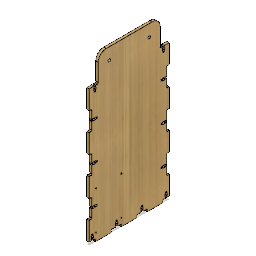
Square-plate-IIIS-power-rev1_8mm v1 (Autodesk Fusion 360 design; units mm, degrees)
Autodesk Fusion 360 part; units mm, degrees
sketch "Basic shape" plane through (0, 0, 0) normal (1, 0, 0) x (0, 0, -1)
  line L0 (-117.75, 0) -> (117.75, 0)
  line L1 (117.75, 0) -> (117.75, 417)
  line L2 (117.75, 417) -> (-117.75, 417)
  line L3 (-117.75, 417) -> (-117.75, 0)
  line L4 (-97.5, 417) -> (97.5, 417)
  line L5 (97.5, 417) -> (97.5, 500)
  line L6 (97.5, 500) -> (-97.5, 500)
  line L7 (-97.5, 500) -> (-97.5, 417)
  line L8 (117.75, 0) -> (125.75, 0)
  line L9 (125.75, 0) -> (125.75, 60)
  line L10 (125.75, 60) -> (117.75, 60)
  line L11 (117.75, 60) -> (117.75, 0)
  line L12 (117.75, 119) -> (125.75, 119)
  line L13 (125.75, 119) -> (125.75, 179)
  line L14 (125.75, 179) -> (117.75, 179)
  line L15 (117.75, 179) -> (117.75, 119)
  line L16 (117.75, 238) -> (125.75, 238)
  line L17 (125.75, 238) -> (125.75, 298)
  line L18 (125.75, 298) -> (117.75, 298)
  line L19 (117.75, 298) -> (117.75, 238)
  line L20 (117.75, 357) -> (125.75, 357)
  line L21 (125.75, 357) -> (125.75, 417)
  line L22 (125.75, 417) -> (117.75, 417)
  line L23 (117.75, 417) -> (117.75, 357)
  curve K0
  line L24 (-55.75, 0) -> (-55.75, -8)
  line L25 (-55.75, -8) -> (-105.75, -8)
  line L26 (-25, 0) -> (25, 0)
  line L27 (25, 0) -> (25, -8)
  line L28 (25, -8) -> (-25, -8)
  line L29 (-25, -8) -> (-25, 0)
  line L30 (117.75, 0) -> (55.75, 0)
  line L31 (55.75, 0) -> (55.75, -8)
  line L32 (55.75, -8) -> (105.75, -8)
  line L33 (-55.75, -8) -> (-25, -8) construction
  line L34 (25, -8) -> (55.75, -8) construction
  line L35 (-117.75, 0) -> (-125.75, 0)
  line L36 (-125.75, 0) -> (-125.75, 60)
  line L37 (-125.75, 60) -> (-117.75, 60)
  line L38 (-117.75, 60) -> (-117.75, 0)
  line L39 (-117.75, 119) -> (-125.75, 119)
  line L40 (-125.75, 119) -> (-125.75, 179)
  line L41 (-125.75, 179) -> (-117.75, 179)
  line L42 (-117.75, 179) -> (-117.75, 119)
  line L43 (-117.75, 238) -> (-125.75, 238)
  line L44 (-125.75, 238) -> (-125.75, 298)
  line L45 (-125.75, 298) -> (-117.75, 298)
  line L46 (-117.75, 298) -> (-117.75, 238)
  line L47 (-117.75, 357) -> (-125.75, 357)
  line L48 (-125.75, 357) -> (-125.75, 417)
  line L49 (-125.75, 417) -> (-117.75, 417)
  line L50 (-117.75, 417) -> (-117.75, 357)
  line L51 (117.75, 60) -> (117.75, 119)
  line L52 (125.75, 60) -> (125.75, 119) construction
  line L53 (125.75, 179) -> (125.75, 238) construction
  line L54 (125.75, 298) -> (125.75, 357) construction
  line L55 (-125.75, 60) -> (-125.75, 119) construction
  line L56 (-125.75, 179) -> (-125.75, 238) construction
  line L57 (-125.75, 357) -> (-125.75, 298) construction
  line L58 (-105.75, -8) -> (-105.75, 0)
  line L59 (105.7775, 0) -> (105.75, -8)
  line L60 (97.5, 417) -> (125.75, 417)
  line L61 (-125.75, 417) -> (-97.5, 417)
  dimension "d1" = 235.5
  dimension "d2" = 417
  dimension "d3" = 83
  dimension "d4" = 195
  dimension "d9" = 60
  dimension "d10" = 60
  dimension "d11" = 60
  dimension "d12" = 60
  dimension "d18" = 50
  dimension "d20" = 8
  dimension "d21" = 8
  dimension "d22" = 60
  dimension "d24" = 60
  dimension "d26" = 60
  dimension "d28" = 60
  dimension "d29" = 8
  dimension "d30" = 8
  dimension "d83" = 20
  dimension "d84" = 8
  dimension "d85" = 20
  dimension "d86" = 25.75
  dimension "d87" = 25.75
  dimension "d363" = 50
  dimension "d364" = 50
  measures "d2" distance of origin
  measures "d22" distance of origin
  measures "d30" distance of origin
  measures "d84" distance of origin
  measures "d85" distance of origin
extrude "Extrude1" add sketch "Basic shape" along normal blind 8
sketch "T slots horizontal" plane through (8, 0, 0) normal (1, 0, 0) x (0, 0, -1)
  line L0 (-117.75, 357) -> (-117.75, 298)
  line L1 (-117.75, 298) -> (-125.75, 298)
  line L2 (-125.75, 298) -> (-125.75, 238)
  line L3 (-125.75, 238) -> (-117.75, 238)
  line L4 (-117.75, 238) -> (-117.75, 179)
  line L5 (-117.75, 179) -> (-125.75, 179)
  line L6 (-125.75, 179) -> (-125.75, 119)
  line L7 (-125.75, 119) -> (-117.75, 119)
  line L8 (-117.75, 119) -> (-117.75, 60)
  line L9 (-117.75, 60) -> (-125.75, 60)
  line L10 (-125.75, 60) -> (-125.75, 0)
  line L11 (-125.75, 0) -> (-117.75, 0)
  line L12 (-105.75, -8) -> (-55.75, -8)
  line L13 (-55.75, -8) -> (-55.75, 0)
  curve K0
  line L14 (-25, 0) -> (-25, -8)
  line L15 (-25, -8) -> (25, -8)
  line L16 (25, -8) -> (25, 0)
  line L17 (25, 0) -> (55.75, 0)
  line L18 (55.75, 0) -> (55.75, -8)
  line L19 (55.75, -8) -> (105.75, -8)
  line L20 (105.7775, 0) -> (125.75, 0)
  line L21 (125.75, 0) -> (125.75, 60)
  line L22 (125.75, 60) -> (117.75, 60)
  line L23 (117.75, 60) -> (117.75, 119)
  line L24 (117.75, 119) -> (125.75, 119)
  line L25 (125.75, 119) -> (125.75, 179)
  line L26 (125.75, 179) -> (117.75, 179)
  line L27 (117.75, 179) -> (117.75, 238)
  line L28 (117.75, 238) -> (125.75, 238)
  line L29 (125.75, 238) -> (125.75, 298)
  line L30 (125.75, 298) -> (117.75, 298)
  line L31 (117.75, 298) -> (117.75, 357)
  line L32 (117.75, 357) -> (125.75, 357)
  line L33 (125.75, 357) -> (125.75, 417)
  line L34 (125.75, 417) -> (97.5, 417)
  line L35 (97.5, 417) -> (97.5, 500)
  line L36 (97.5, 500) -> (-97.5, 500)
  line L37 (-97.5, 500) -> (-97.5, 417)
  line L38 (-97.5, 417) -> (-125.75, 417)
  line L39 (-125.75, 417) -> (-125.75, 357)
  line L40 (-125.75, 357) -> (-117.75, 357)
  line L41 (-41.885, 0) -> (-37.865, 0)
  line L42 (-37.865, 0) -> (-37.865, 17.5)
  line L43 (-37.865, 17.5) -> (-41.885, 17.5)
  line L44 (-41.885, 17.5) -> (-41.885, 0)
  line L45 (-43.355, 12.5) -> (-36.355, 12.5)
  line L46 (-36.355, 12.5) -> (-36.355, 5)
  line L47 (-36.355, 5) -> (-43.355, 5)
  line L48 (-43.355, 5) -> (-43.355, 12.5)
  line L49 (-109.635, 417) -> (-105.615, 417)
  line L50 (-105.615, 417) -> (-105.615, 399.5)
  line L51 (-105.615, 399.5) -> (-109.635, 399.5)
  line L52 (-109.635, 399.5) -> (-109.635, 417)
  line L53 (-111.105, 412) -> (-104.105, 412)
  line L54 (-104.105, 412) -> (-104.105, 404.5)
  line L55 (-104.105, 404.5) -> (-111.105, 404.5)
  line L56 (-111.105, 404.5) -> (-111.105, 412)
  line L57 (-113.74, 0) -> (-113.74, 17.5)
  line L58 (-117.76, 17.5) -> (-117.76, 0)
  line L59 (-113.74, 17.5) -> (-117.76, 17.5)
  line L60 (-119.23, 5) -> (-119.23, 12.5)
  line L61 (-112.23, 5) -> (-119.23, 5)
  line L62 (-117.76, 0) -> (-113.74, 0)
  line L63 (-112.23, 12.5) -> (-112.23, 5)
  line L64 (-119.23, 12.5) -> (-112.23, 12.5)
  line L65 (-105.75, 0) -> (-105.75, -8)
  line L66 (105.75, -8) -> (105.7775, 0)
  line L67 (-55.75, 0) -> (-25, 0)
  dimension "d31" = 4.02
  dimension "d32" = 7
  dimension "d33" = 1.51
  dimension "d34" = 5
  dimension "d35" = 17.5
  dimension "d36" = 7.5
  dimension "d37" = 4.02
  dimension "d38" = 17.5
  dimension "d39" = 7.5
  dimension "d40" = 1.51
  dimension "d41" = 7
  dimension "d42" = 5
  dimension "d66" = 4.02
  dimension "d67" = 7
  dimension "d68" = 1.51
  dimension "d70" = 17.5
  dimension "d71" = 7.5
  dimension "d81" = 10.125
  dimension "d89" = 12.875
  dimension "d93" = 5
  dimension "d95" = 10
  measures "d33" distance of L42
  measures "d68" distance of L57
  measures "d70" distance of origin
  measures "d89" distance of origin
  measures "d93" distance of origin
  measures "d95" distance of origin L65
extrude "Extrude2" cut sketch "T slots horizontal" against normal through all
mirror "Mirror1" about plane through (0, 0, 0) normal (0, 0, 1) of "Extrude2"
sketch "T slots vertical" plane through (8, 0, 0) normal (1, 0, 0) x (0, 0, -1)
  line L0 (37.865, 0) -> (37.865, 5)
  line L1 (37.865, 5) -> (36.355, 5)
  line L2 (36.355, 5) -> (36.355, 12.5)
  line L3 (36.355, 12.5) -> (37.865, 12.5)
  line L4 (37.865, 12.5) -> (37.865, 17.5)
  line L5 (37.865, 17.5) -> (41.885, 17.5)
  line L6 (41.885, 17.5) -> (41.885, 12.5)
  line L7 (41.885, 12.5) -> (43.355, 12.5)
  line L8 (55.75, 0) -> (55.75, -8)
  line L9 (55.75, -8) -> (105.75, -8)
  line L10 (105.7775, 0) -> (113.74, 0)
  line L11 (125.75, 0) -> (125.75, 60)
  line L12 (125.75, 60) -> (117.75, 60)
  line L13 (117.75, 60) -> (117.75, 119)
  line L14 (117.75, 119) -> (125.75, 119)
  line L15 (125.75, 119) -> (125.75, 179)
  line L16 (125.75, 179) -> (117.75, 179)
  line L17 (117.75, 179) -> (117.75, 238)
  line L18 (117.75, 238) -> (125.75, 238)
  line L19 (125.75, 238) -> (125.75, 298)
  line L20 (125.75, 298) -> (117.75, 298)
  line L21 (117.75, 298) -> (117.75, 357)
  line L22 (117.75, 357) -> (125.75, 357)
  line L23 (125.75, 357) -> (125.75, 417)
  line L24 (125.75, 417) -> (109.635, 417)
  line L25 (109.635, 417) -> (109.635, 412)
  line L26 (109.635, 412) -> (111.105, 412)
  line L27 (111.105, 412) -> (111.105, 404.5)
  line L28 (111.105, 404.5) -> (109.635, 404.5)
  line L29 (109.635, 404.5) -> (109.635, 399.5)
  line L30 (109.635, 399.5) -> (105.615, 399.5)
  line L31 (105.615, 399.5) -> (105.615, 404.5)
  line L32 (105.615, 404.5) -> (104.105, 404.5)
  line L33 (104.105, 404.5) -> (104.105, 412)
  line L34 (104.105, 412) -> (105.615, 412)
  line L35 (105.615, 412) -> (105.615, 417)
  line L36 (105.615, 417) -> (97.5, 417)
  line L37 (97.5, 417) -> (97.5, 500)
  line L38 (97.5, 500) -> (-97.5, 500)
  line L39 (-97.5, 500) -> (-97.5, 417)
  line L40 (-97.5, 417) -> (-105.615, 417)
  line L41 (-105.615, 417) -> (-105.615, 412)
  line L42 (-105.615, 412) -> (-104.105, 412)
  line L43 (-104.105, 412) -> (-104.105, 404.5)
  line L44 (-104.105, 404.5) -> (-105.615, 404.5)
  line L45 (-105.615, 404.5) -> (-105.615, 399.5)
  line L46 (-105.615, 399.5) -> (-109.635, 399.5)
  line L47 (-109.635, 399.5) -> (-109.635, 404.5)
  line L48 (-109.635, 404.5) -> (-111.105, 404.5)
  line L49 (-111.105, 404.5) -> (-111.105, 412)
  line L50 (-111.105, 412) -> (-109.635, 412)
  line L51 (-109.635, 412) -> (-109.635, 417)
  line L52 (-109.635, 417) -> (-125.75, 417)
  line L53 (-125.75, 417) -> (-125.75, 357)
  line L54 (-125.75, 357) -> (-117.75, 357)
  line L55 (-117.75, 357) -> (-117.75, 298)
  line L56 (-117.75, 298) -> (-125.75, 298)
  line L57 (-125.75, 298) -> (-125.75, 238)
  line L58 (-125.75, 238) -> (-117.75, 238)
  line L59 (-117.75, 238) -> (-117.75, 179)
  line L60 (-117.75, 179) -> (-125.75, 179)
  line L61 (-125.75, 179) -> (-125.75, 119)
  line L62 (-125.75, 119) -> (-117.75, 119)
  line L63 (-117.75, 119) -> (-117.75, 60)
  line L64 (-117.75, 60) -> (-125.75, 60)
  line L65 (-125.75, 60) -> (-125.75, 0)
  line L66 (-125.75, 0) -> (-117.76, 0)
  line L67 (-105.75, -8) -> (-55.75, -8)
  line L68 (-55.75, -8) -> (-55.75, 0)
  line L69 (41.885, 0) -> (55.75, 0)
  line L70 (-43.355, 12.5) -> (-41.885, 12.5)
  line L71 (-41.885, 12.5) -> (-41.885, 17.5)
  line L72 (-41.885, 17.5) -> (-37.865, 17.5)
  line L73 (-37.865, 17.5) -> (-37.865, 12.5)
  line L74 (-37.865, 12.5) -> (-36.355, 12.5)
  line L75 (-36.355, 12.5) -> (-36.355, 5)
  line L76 (-36.355, 5) -> (-37.865, 5)
  line L77 (-37.865, 5) -> (-37.865, 0)
  line L78 (-37.865, 0) -> (-25, 0)
  line L79 (-25, 0) -> (-25, -8)
  line L80 (-25, -8) -> (25, -8)
  line L81 (25, -8) -> (25, 0)
  line L82 (25, 0) -> (37.865, 0)
  line L83 (-117.75, 91.51) -> (-100.25, 91.51)
  line L84 (-100.25, 91.51) -> (-100.25, 87.49)
  line L85 (-100.25, 87.49) -> (-117.75, 87.49)
  line L86 (-117.75, 87.49) -> (-117.75, 91.51)
  line L87 (-112.75, 93.02) -> (-105.25, 93.02)
  line L88 (-105.25, 93.02) -> (-105.25, 86.02)
  line L89 (-105.25, 86.02) -> (-112.75, 86.02)
  line L90 (-112.75, 86.02) -> (-112.75, 93.02)
  line L91 (113.74, 12.5) -> (113.74, 17.5)
  line L92 (113.74, 17.5) -> (117.76, 17.5)
  line L93 (117.76, 17.5) -> (117.76, 12.5)
  line L94 (117.76, 12.5) -> (119.23, 12.5)
  line L95 (119.23, 12.5) -> (119.23, 5)
  line L96 (119.23, 5) -> (117.76, 5)
  line L97 (117.76, 5) -> (117.76, 0)
  line L98 (117.76, 0) -> (125.75, 0)
  line L99 (-117.76, 0) -> (-117.76, 5)
  line L100 (-117.76, 5) -> (-119.23, 5)
  line L101 (-119.23, 5) -> (-119.23, 12.5)
  line L102 (-119.23, 12.5) -> (-117.76, 12.5)
  line L103 (-117.76, 12.5) -> (-117.76, 17.5)
  line L104 (-117.76, 17.5) -> (-113.74, 17.5)
  line L105 (-113.74, 17.5) -> (-113.74, 12.5)
  line L106 (-105.75, 0) -> (-105.75, -8)
  line L107 (105.75, -8) -> (105.7775, 0)
  line L108 (43.355, 12.5) -> (43.355, 5)
  line L109 (43.355, 5) -> (41.885, 5)
  line L110 (41.885, 5) -> (41.885, 0)
  line L111 (113.74, 0) -> (113.74, 5)
  line L112 (113.74, 5) -> (112.23, 5)
  line L113 (112.23, 5) -> (112.23, 12.5)
  line L114 (112.23, 12.5) -> (113.74, 12.5)
  line L115 (-113.74, 12.5) -> (-112.23, 12.5)
  line L116 (-112.23, 12.5) -> (-112.23, 5)
  line L117 (-112.23, 5) -> (-113.74, 5)
  line L118 (-113.74, 5) -> (-113.74, 0)
  line L119 (-41.885, 0) -> (-41.885, 5)
  line L120 (-41.885, 5) -> (-43.355, 5)
  line L121 (-43.355, 5) -> (-43.355, 12.5)
  line L122 (-113.74, 0) -> (-105.75, 0)
  line L123 (-55.75, 0) -> (-41.885, 0)
  dimension "d45" = 1.51
  dimension "d46" = 4.02
  dimension "d47" = 7
  dimension "d48" = 7.5
  dimension "d49" = 5
  dimension "d50" = 17.5
  dimension "d94" = 2
extrude "Extrude3" cut sketch "T slots vertical" against normal through all contours L63 L83 L85 L86 L90 | L83 L85 L88 L90 | L85 L88 L89 L90 | L83 L87 L88 L90 | L83 L84 L85 L88
pattern_linear "R-Pattern1" count 3 spacing 118.6667 along (0, 1, 0) of "Extrude3"
mirror "Mirror2" about plane through (0, 0, 0) normal (0, 0, 1) of "Extrude3", "R-Pattern1"
fillet "Fillet1" radius 25 2 edges at (4, 500, -97.5) (4, 500, 97.5)
sketch "Bar holder" plane through (8, 0, 0) normal (1, 0, 0) x (0, 0, -1)
  arc A0 (-72.5, 500) -> (-97.5, 475) centre (-72.5, 475) ccw
  line L0 (-97.5, 475) -> (-97.5, 417)
  line L1 (-97.5, 417) -> (-105.615, 417)
  line L2 (-105.615, 417) -> (-105.615, 412)
  line L3 (-105.615, 412) -> (-104.105, 412)
  line L4 (-104.105, 412) -> (-104.105, 404.5)
  line L5 (-104.105, 404.5) -> (-105.615, 404.5)
  line L6 (-105.615, 404.5) -> (-105.615, 399.5)
  line L7 (-105.615, 399.5) -> (-109.635, 399.5)
  line L8 (-109.635, 399.5) -> (-109.635, 404.5)
  line L9 (-109.635, 404.5) -> (-111.105, 404.5)
  line L10 (-111.105, 404.5) -> (-111.105, 412)
  line L11 (-111.105, 412) -> (-109.635, 412)
  line L12 (-109.635, 412) -> (-109.635, 417)
  line L13 (-109.635, 417) -> (-125.75, 417)
  line L14 (-125.75, 417) -> (-125.75, 357)
  line L15 (-125.75, 357) -> (-117.75, 357)
  line L16 (-117.75, 357) -> (-117.75, 328.8433)
  line L17 (-117.75, 328.8433) -> (-112.75, 328.8433)
  line L18 (-112.75, 328.8433) -> (-112.75, 330.3533)
  line L19 (-112.75, 330.3533) -> (-105.25, 330.3533)
  line L20 (-105.25, 330.3533) -> (-105.25, 328.8433)
  line L21 (-105.25, 328.8433) -> (-100.25, 328.8433)
  line L22 (-100.25, 328.8433) -> (-100.25, 324.8233)
  line L23 (-100.25, 324.8233) -> (-105.25, 324.8233)
  line L24 (-105.25, 324.8233) -> (-105.25, 323.3533)
  line L25 (-105.25, 323.3533) -> (-112.75, 323.3533)
  line L26 (-112.75, 323.3533) -> (-112.75, 324.8233)
  line L27 (-112.75, 324.8233) -> (-117.75, 324.8233)
  line L28 (-117.75, 324.8233) -> (-117.75, 298)
  line L29 (-117.75, 298) -> (-125.75, 298)
  line L30 (-125.75, 298) -> (-125.75, 238)
  line L31 (-125.75, 238) -> (-117.75, 238)
  line L32 (-117.75, 238) -> (-117.75, 210.1767)
  line L33 (-117.75, 210.1767) -> (-112.75, 210.1767)
  line L34 (-112.75, 210.1767) -> (-112.75, 211.6867)
  line L35 (-112.75, 211.6867) -> (-105.25, 211.6867)
  line L36 (-105.25, 211.6867) -> (-105.25, 210.1767)
  line L37 (-105.25, 210.1767) -> (-100.25, 210.1767)
  line L38 (-100.25, 210.1767) -> (-100.25, 206.1567)
  line L39 (-100.25, 206.1567) -> (-105.25, 206.1567)
  line L40 (-105.25, 206.1567) -> (-105.25, 204.6867)
  line L41 (-105.25, 204.6867) -> (-112.75, 204.6867)
  line L42 (-112.75, 204.6867) -> (-112.75, 206.1567)
  line L43 (-112.75, 206.1567) -> (-117.75, 206.1567)
  line L44 (-117.75, 206.1567) -> (-117.75, 179)
  line L45 (-117.75, 179) -> (-125.75, 179)
  line L46 (-125.75, 179) -> (-125.75, 119)
  line L47 (-125.75, 119) -> (-117.75, 119)
  line L48 (-117.75, 119) -> (-117.75, 91.51)
  line L49 (-117.75, 91.51) -> (-112.75, 91.51)
  line L50 (-112.75, 91.51) -> (-112.75, 93.02)
  line L51 (-112.75, 93.02) -> (-105.25, 93.02)
  line L52 (-105.25, 93.02) -> (-105.25, 91.51)
  line L53 (-105.25, 91.51) -> (-100.25, 91.51)
  line L54 (-100.25, 91.51) -> (-100.25, 87.49)
  line L55 (-100.25, 87.49) -> (-105.25, 87.49)
  line L56 (-105.25, 87.49) -> (-105.25, 86.02)
  line L57 (-105.25, 86.02) -> (-112.75, 86.02)
  line L58 (-112.75, 86.02) -> (-112.75, 87.49)
  line L59 (-112.75, 87.49) -> (-117.75, 87.49)
  line L60 (-117.75, 87.49) -> (-117.75, 60)
  line L61 (-117.75, 60) -> (-125.75, 60)
  line L62 (-125.75, 60) -> (-125.75, 0)
  line L63 (-125.75, 0) -> (-117.76, 0)
  line L64 (-105.75, -8) -> (-55.75, -8)
  line L65 (-55.75, -8) -> (-55.75, 0)
  line L66 (-55.75, 0) -> (-41.885, 0)
  line L67 (-43.355, 12.5) -> (-41.885, 12.5)
  line L68 (-41.885, 12.5) -> (-41.885, 17.5)
  line L69 (-41.885, 17.5) -> (-37.865, 17.5)
  line L70 (-37.865, 17.5) -> (-37.865, 12.5)
  line L71 (-37.865, 12.5) -> (-36.355, 12.5)
  line L72 (-36.355, 12.5) -> (-36.355, 5)
  line L73 (-36.355, 5) -> (-37.865, 5)
  line L74 (-37.865, 5) -> (-37.865, 0)
  line L75 (-37.865, 0) -> (-25, 0)
  line L76 (-25, 0) -> (-25, -8)
  line L77 (-25, -8) -> (25, -8)
  line L78 (25, -8) -> (25, 0)
  line L79 (25, 0) -> (37.865, 0)
  line L80 (37.865, 0) -> (37.865, 5)
  line L81 (37.865, 5) -> (36.355, 5)
  line L82 (36.355, 5) -> (36.355, 12.5)
  line L83 (36.355, 12.5) -> (37.865, 12.5)
  line L84 (37.865, 12.5) -> (37.865, 17.5)
  line L85 (37.865, 17.5) -> (41.885, 17.5)
  line L86 (41.885, 17.5) -> (41.885, 12.5)
  line L87 (41.885, 12.5) -> (43.355, 12.5)
  line L88 (55.75, 0) -> (55.75, -8)
  line L89 (55.75, -8) -> (105.75, -8)
  line L90 (105.7775, 0) -> (113.74, 0)
  line L91 (125.75, 0) -> (125.75, 60)
  line L92 (125.75, 60) -> (117.75, 60)
  line L93 (117.75, 60) -> (117.75, 87.49)
  line L94 (117.75, 87.49) -> (112.75, 87.49)
  line L95 (112.75, 87.49) -> (112.75, 86.02)
  line L96 (112.75, 86.02) -> (105.25, 86.02)
  line L97 (105.25, 86.02) -> (105.25, 87.49)
  line L98 (105.25, 87.49) -> (100.25, 87.49)
  line L99 (100.25, 87.49) -> (100.25, 91.51)
  line L100 (100.25, 91.51) -> (105.25, 91.51)
  line L101 (105.25, 91.51) -> (105.25, 93.02)
  line L102 (105.25, 93.02) -> (112.75, 93.02)
  line L103 (112.75, 93.02) -> (112.75, 91.51)
  line L104 (112.75, 91.51) -> (117.75, 91.51)
  line L105 (117.75, 91.51) -> (117.75, 119)
  line L106 (117.75, 119) -> (125.75, 119)
  line L107 (125.75, 119) -> (125.75, 179)
  line L108 (125.75, 179) -> (117.75, 179)
  line L109 (117.75, 179) -> (117.75, 206.1567)
  line L110 (117.75, 206.1567) -> (112.75, 206.1567)
  line L111 (112.75, 206.1567) -> (112.75, 204.6867)
  line L112 (112.75, 204.6867) -> (105.25, 204.6867)
  line L113 (105.25, 204.6867) -> (105.25, 206.1567)
  line L114 (105.25, 206.1567) -> (100.25, 206.1567)
  line L115 (100.25, 206.1567) -> (100.25, 210.1767)
  line L116 (100.25, 210.1767) -> (105.25, 210.1767)
  line L117 (105.25, 210.1767) -> (105.25, 211.6867)
  line L118 (105.25, 211.6867) -> (112.75, 211.6867)
  line L119 (112.75, 211.6867) -> (112.75, 210.1767)
  line L120 (112.75, 210.1767) -> (117.75, 210.1767)
  line L121 (117.75, 210.1767) -> (117.75, 238)
  line L122 (117.75, 238) -> (125.75, 238)
  line L123 (125.75, 238) -> (125.75, 298)
  line L124 (125.75, 298) -> (117.75, 298)
  line L125 (117.75, 298) -> (117.75, 324.8233)
  line L126 (117.75, 324.8233) -> (112.75, 324.8233)
  line L127 (112.75, 324.8233) -> (112.75, 323.3533)
  line L128 (112.75, 323.3533) -> (105.25, 323.3533)
  line L129 (105.25, 323.3533) -> (105.25, 324.8233)
  line L130 (105.25, 324.8233) -> (100.25, 324.8233)
  line L131 (100.25, 324.8233) -> (100.25, 328.8433)
  line L132 (100.25, 328.8433) -> (105.25, 328.8433)
  line L133 (105.25, 328.8433) -> (105.25, 330.3533)
  line L134 (105.25, 330.3533) -> (112.75, 330.3533)
  line L135 (112.75, 330.3533) -> (112.75, 328.8433)
  line L136 (112.75, 328.8433) -> (117.75, 328.8433)
  line L137 (117.75, 328.8433) -> (117.75, 357)
  line L138 (117.75, 357) -> (125.75, 357)
  line L139 (125.75, 357) -> (125.75, 417)
  line L140 (125.75, 417) -> (109.635, 417)
  line L141 (109.635, 417) -> (109.635, 412)
  line L142 (109.635, 412) -> (111.105, 412)
  line L143 (111.105, 412) -> (111.105, 404.5)
  line L144 (111.105, 404.5) -> (109.635, 404.5)
  line L145 (109.635, 404.5) -> (109.635, 399.5)
  line L146 (109.635, 399.5) -> (105.615, 399.5)
  line L147 (105.615, 399.5) -> (105.615, 404.5)
  line L148 (105.615, 404.5) -> (104.105, 404.5)
  line L149 (104.105, 404.5) -> (104.105, 412)
  line L150 (104.105, 412) -> (105.615, 412)
  line L151 (105.615, 412) -> (105.615, 417)
  line L152 (105.615, 417) -> (97.5, 417)
  line L153 (97.5, 417) -> (97.5, 475)
  arc A1 (97.5, 475) -> (72.5, 500) centre (72.5, 475) ccw
  line L154 (72.5, 500) -> (-72.5, 500)
  line L155 (-62.5, 462.5) -> (62.5, 462.5) construction
  circle A2 centre (-62.5, 462.5) radius 4
  circle A3 centre (62.5, 462.5) radius 4
  line L156 (0, 500) -> (0, 417) construction
  line L157 (-97.5, 417) -> (97.5, 417) construction
  line L158 (-97.5, 427) -> (97.5, 427) construction
  line L159 (-117.76, 0) -> (-117.76, 5)
  line L160 (-117.76, 5) -> (-119.23, 5)
  line L161 (-119.23, 5) -> (-119.23, 12.5)
  line L162 (-119.23, 12.5) -> (-117.76, 12.5)
  line L163 (-117.76, 12.5) -> (-117.76, 17.5)
  line L164 (-117.76, 17.5) -> (-113.74, 17.5)
  line L165 (-113.74, 17.5) -> (-113.74, 12.5)
  line L166 (113.74, 12.5) -> (113.74, 17.5)
  line L167 (113.74, 17.5) -> (117.76, 17.5)
  line L168 (117.76, 17.5) -> (117.76, 12.5)
  line L169 (117.76, 12.5) -> (119.23, 12.5)
  line L170 (119.23, 12.5) -> (119.23, 5)
  line L171 (119.23, 5) -> (117.76, 5)
  line L172 (117.76, 5) -> (117.76, 0)
  line L173 (117.76, 0) -> (125.75, 0)
  line L174 (-105.75, 0) -> (-105.75, -8)
  line L175 (105.75, -8) -> (105.7775, 0)
  line L176 (-113.74, 12.5) -> (-112.23, 12.5)
  line L177 (-112.23, 12.5) -> (-112.23, 5)
  line L178 (-112.23, 5) -> (-113.74, 5)
  line L179 (-113.74, 5) -> (-113.74, 0)
  line L180 (-41.885, 0) -> (-41.885, 5)
  line L181 (-41.885, 5) -> (-43.355, 5)
  line L182 (-43.355, 5) -> (-43.355, 12.5)
  line L183 (43.355, 12.5) -> (43.355, 5)
  line L184 (43.355, 5) -> (41.885, 5)
  line L185 (41.885, 5) -> (41.885, 0)
  line L186 (41.885, 0) -> (55.75, 0)
  line L187 (113.74, 0) -> (113.74, 5)
  line L188 (113.74, 5) -> (112.23, 5)
  line L189 (112.23, 5) -> (112.23, 12.5)
  line L190 (112.23, 12.5) -> (113.74, 12.5)
  line L191 (-113.74, 0) -> (-105.75, 0)
  dimension "d58" = 125
  dimension "d59" = 8
  dimension "d60" = 8
  dimension "d62" = 10
  dimension "d63" = 75
  dimension "d64" = 37.5
  measures "d59" diameter of A2
  measures "d60" diameter of A3
  measures "d62" distance of L157 L158
  measures "d63" distance of L154 L158
  measures "d64" distance of L154
extrude "Extrude4" cut sketch "Bar holder" against normal through all contours A2 | A3
sketch "Power holes" plane through (8, 0, 0) normal (1, 0, 0) x (0, 0, -1)
  circle A0 centre (-62.5, 462.5) radius 4
  circle A1 centre (62.5, 462.5) radius 4
  arc A2 (-72.5, 500) -> (-97.5, 475) centre (-72.5, 475) ccw
  line L0 (-97.5, 475) -> (-97.5, 417)
  line L1 (-97.5, 417) -> (-105.615, 417)
  line L2 (-105.615, 417) -> (-105.615, 412)
  line L3 (-105.615, 412) -> (-104.105, 412)
  line L4 (-104.105, 412) -> (-104.105, 404.5)
  line L5 (-104.105, 404.5) -> (-105.615, 404.5)
  line L6 (-105.615, 404.5) -> (-105.615, 399.5)
  line L7 (-105.615, 399.5) -> (-109.635, 399.5)
  line L8 (-109.635, 399.5) -> (-109.635, 404.5)
  line L9 (-109.635, 404.5) -> (-111.105, 404.5)
  line L10 (-111.105, 404.5) -> (-111.105, 412)
  line L11 (-111.105, 412) -> (-109.635, 412)
  line L12 (-109.635, 412) -> (-109.635, 417)
  line L13 (-109.635, 417) -> (-125.75, 417)
  line L14 (-125.75, 417) -> (-125.75, 357)
  line L15 (-125.75, 357) -> (-117.75, 357)
  line L16 (-117.75, 357) -> (-117.75, 328.8433)
  line L17 (-117.75, 328.8433) -> (-112.75, 328.8433)
  line L18 (-112.75, 328.8433) -> (-112.75, 330.3533)
  line L19 (-112.75, 330.3533) -> (-105.25, 330.3533)
  line L20 (-105.25, 330.3533) -> (-105.25, 328.8433)
  line L21 (-105.25, 328.8433) -> (-100.25, 328.8433)
  line L22 (-100.25, 328.8433) -> (-100.25, 324.8233)
  line L23 (-100.25, 324.8233) -> (-105.25, 324.8233)
  line L24 (-105.25, 324.8233) -> (-105.25, 323.3533)
  line L25 (-105.25, 323.3533) -> (-112.75, 323.3533)
  line L26 (-112.75, 323.3533) -> (-112.75, 324.8233)
  line L27 (-112.75, 324.8233) -> (-117.75, 324.8233)
  line L28 (-117.75, 324.8233) -> (-117.75, 298)
  line L29 (-117.75, 298) -> (-125.75, 298)
  line L30 (-125.75, 298) -> (-125.75, 238)
  line L31 (-125.75, 238) -> (-117.75, 238)
  line L32 (-117.75, 238) -> (-117.75, 210.1767)
  line L33 (-117.75, 210.1767) -> (-112.75, 210.1767)
  line L34 (-112.75, 210.1767) -> (-112.75, 211.6867)
  line L35 (-112.75, 211.6867) -> (-105.25, 211.6867)
  line L36 (-105.25, 211.6867) -> (-105.25, 210.1767)
  line L37 (-105.25, 210.1767) -> (-100.25, 210.1767)
  line L38 (-100.25, 210.1767) -> (-100.25, 206.1567)
  line L39 (-100.25, 206.1567) -> (-105.25, 206.1567)
  line L40 (-105.25, 206.1567) -> (-105.25, 204.6867)
  line L41 (-105.25, 204.6867) -> (-112.75, 204.6867)
  line L42 (-112.75, 204.6867) -> (-112.75, 206.1567)
  line L43 (-112.75, 206.1567) -> (-117.75, 206.1567)
  line L44 (-117.75, 206.1567) -> (-117.75, 179)
  line L45 (-117.75, 179) -> (-125.75, 179)
  line L46 (-125.75, 179) -> (-125.75, 119)
  line L47 (-125.75, 119) -> (-117.75, 119)
  line L48 (-117.75, 119) -> (-117.75, 91.51)
  line L49 (-117.75, 91.51) -> (-112.75, 91.51)
  line L50 (-112.75, 91.51) -> (-112.75, 93.02)
  line L51 (-112.75, 93.02) -> (-105.25, 93.02)
  line L52 (-105.25, 93.02) -> (-105.25, 91.51)
  line L53 (-105.25, 91.51) -> (-100.25, 91.51)
  line L54 (-100.25, 91.51) -> (-100.25, 87.49)
  line L55 (-100.25, 87.49) -> (-105.25, 87.49)
  line L56 (-105.25, 87.49) -> (-105.25, 86.02)
  line L57 (-105.25, 86.02) -> (-112.75, 86.02)
  line L58 (-112.75, 86.02) -> (-112.75, 87.49)
  line L59 (-112.75, 87.49) -> (-117.75, 87.49)
  line L60 (-117.75, 87.49) -> (-117.75, 60)
  line L61 (-117.75, 60) -> (-125.75, 60)
  line L62 (-125.75, 60) -> (-125.75, 0)
  line L63 (-125.75, 0) -> (-117.76, 0)
  line L64 (-117.76, 0) -> (-117.76, 5)
  line L65 (-117.76, 5) -> (-119.23, 5)
  line L66 (-119.23, 5) -> (-119.23, 12.5)
  line L67 (-119.23, 12.5) -> (-117.76, 12.5)
  line L68 (-117.76, 12.5) -> (-117.76, 17.5)
  line L69 (-117.76, 17.5) -> (-113.74, 17.5)
  line L70 (-113.74, 17.5) -> (-113.74, 12.5)
  line L71 (-105.75, -8) -> (-55.75, -8)
  line L72 (-55.75, -8) -> (-55.75, 0)
  line L73 (-55.75, 0) -> (-41.885, 0)
  line L74 (-43.355, 12.5) -> (-41.885, 12.5)
  line L75 (-41.885, 12.5) -> (-41.885, 17.5)
  line L76 (-41.885, 17.5) -> (-37.865, 17.5)
  line L77 (-37.865, 17.5) -> (-37.865, 12.5)
  line L78 (-37.865, 12.5) -> (-36.355, 12.5)
  line L79 (-36.355, 12.5) -> (-36.355, 5)
  line L80 (-36.355, 5) -> (-37.865, 5)
  line L81 (-37.865, 5) -> (-37.865, 0)
  line L82 (-37.865, 0) -> (-25, 0)
  line L83 (-25, 0) -> (-25, -8)
  line L84 (-25, -8) -> (25, -8)
  line L85 (25, -8) -> (25, 0)
  line L86 (25, 0) -> (37.865, 0)
  line L87 (37.865, 0) -> (37.865, 5)
  line L88 (37.865, 5) -> (36.355, 5)
  line L89 (36.355, 5) -> (36.355, 12.5)
  line L90 (36.355, 12.5) -> (37.865, 12.5)
  line L91 (37.865, 12.5) -> (37.865, 17.5)
  line L92 (37.865, 17.5) -> (41.885, 17.5)
  line L93 (41.885, 17.5) -> (41.885, 12.5)
  line L94 (41.885, 12.5) -> (43.355, 12.5)
  line L95 (55.75, 0) -> (55.75, -8)
  line L96 (55.75, -8) -> (105.75, -8)
  line L97 (105.7775, 0) -> (113.74, 0)
  line L98 (113.74, 12.5) -> (113.74, 17.5)
  line L99 (113.74, 17.5) -> (117.76, 17.5)
  line L100 (117.76, 17.5) -> (117.76, 12.5)
  line L101 (117.76, 12.5) -> (119.23, 12.5)
  line L102 (119.23, 12.5) -> (119.23, 5)
  line L103 (119.23, 5) -> (117.76, 5)
  line L104 (117.76, 5) -> (117.76, 0)
  line L105 (117.76, 0) -> (125.75, 0)
  line L106 (125.75, 0) -> (125.75, 60)
  line L107 (125.75, 60) -> (117.75, 60)
  line L108 (117.75, 60) -> (117.75, 87.49)
  line L109 (117.75, 87.49) -> (112.75, 87.49)
  line L110 (112.75, 87.49) -> (112.75, 86.02)
  line L111 (112.75, 86.02) -> (105.25, 86.02)
  line L112 (105.25, 86.02) -> (105.25, 87.49)
  line L113 (105.25, 87.49) -> (100.25, 87.49)
  line L114 (100.25, 87.49) -> (100.25, 91.51)
  line L115 (100.25, 91.51) -> (105.25, 91.51)
  line L116 (105.25, 91.51) -> (105.25, 93.02)
  line L117 (105.25, 93.02) -> (112.75, 93.02)
  line L118 (112.75, 93.02) -> (112.75, 91.51)
  line L119 (112.75, 91.51) -> (117.75, 91.51)
  line L120 (117.75, 91.51) -> (117.75, 119)
  line L121 (117.75, 119) -> (125.75, 119)
  line L122 (125.75, 119) -> (125.75, 179)
  line L123 (125.75, 179) -> (117.75, 179)
  line L124 (117.75, 179) -> (117.75, 206.1567)
  line L125 (117.75, 206.1567) -> (112.75, 206.1567)
  line L126 (112.75, 206.1567) -> (112.75, 204.6867)
  line L127 (112.75, 204.6867) -> (105.25, 204.6867)
  line L128 (105.25, 204.6867) -> (105.25, 206.1567)
  line L129 (105.25, 206.1567) -> (100.25, 206.1567)
  line L130 (100.25, 206.1567) -> (100.25, 210.1767)
  line L131 (100.25, 210.1767) -> (105.25, 210.1767)
  line L132 (105.25, 210.1767) -> (105.25, 211.6867)
  line L133 (105.25, 211.6867) -> (112.75, 211.6867)
  line L134 (112.75, 211.6867) -> (112.75, 210.1767)
  line L135 (112.75, 210.1767) -> (117.75, 210.1767)
  line L136 (117.75, 210.1767) -> (117.75, 238)
  line L137 (117.75, 238) -> (125.75, 238)
  line L138 (125.75, 238) -> (125.75, 298)
  line L139 (125.75, 298) -> (117.75, 298)
  line L140 (117.75, 298) -> (117.75, 324.8233)
  line L141 (117.75, 324.8233) -> (112.75, 324.8233)
  line L142 (112.75, 324.8233) -> (112.75, 323.3533)
  line L143 (112.75, 323.3533) -> (105.25, 323.3533)
  line L144 (105.25, 323.3533) -> (105.25, 324.8233)
  line L145 (105.25, 324.8233) -> (100.25, 324.8233)
  line L146 (100.25, 324.8233) -> (100.25, 328.8433)
  line L147 (100.25, 328.8433) -> (105.25, 328.8433)
  line L148 (105.25, 328.8433) -> (105.25, 330.3533)
  line L149 (105.25, 330.3533) -> (112.75, 330.3533)
  line L150 (112.75, 330.3533) -> (112.75, 328.8433)
  line L151 (112.75, 328.8433) -> (117.75, 328.8433)
  line L152 (117.75, 328.8433) -> (117.75, 357)
  line L153 (117.75, 357) -> (125.75, 357)
  line L154 (125.75, 357) -> (125.75, 417)
  line L155 (125.75, 417) -> (109.635, 417)
  line L156 (109.635, 417) -> (109.635, 412)
  line L157 (109.635, 412) -> (111.105, 412)
  line L158 (111.105, 412) -> (111.105, 404.5)
  line L159 (111.105, 404.5) -> (109.635, 404.5)
  line L160 (109.635, 404.5) -> (109.635, 399.5)
  line L161 (109.635, 399.5) -> (105.615, 399.5)
  line L162 (105.615, 399.5) -> (105.615, 404.5)
  line L163 (105.615, 404.5) -> (104.105, 404.5)
  line L164 (104.105, 404.5) -> (104.105, 412)
  line L165 (104.105, 412) -> (105.615, 412)
  line L166 (105.615, 412) -> (105.615, 417)
  line L167 (105.615, 417) -> (97.5, 417)
  line L168 (97.5, 417) -> (97.5, 475)
  arc A3 (97.5, 475) -> (72.5, 500) centre (72.5, 475) ccw
  line L169 (72.5, 500) -> (-72.5, 500)
  line L170 (-104.75, 136.75) -> (-24.75, 136.75) construction
  line L171 (-24.75, 136.75) -> (-24.75, 16.75) construction
  line L172 (-24.75, 16.75) -> (-104.75, 16.75) construction
  line L173 (-104.75, 16.75) -> (-104.75, 136.75) construction
  circle A4 centre (-104.75, 136.75) radius 2
  circle A5 centre (-24.75, 136.75) radius 2
  circle A6 centre (-104.75, 16.75) radius 2
  circle A7 centre (-24.75, 16.75) radius 2
  line L174 (-105.75, 0) -> (-105.75, -8)
  line L175 (105.75, -8) -> (105.7775, 0)
  line L176 (-113.74, 12.5) -> (-112.23, 12.5)
  line L177 (-112.23, 12.5) -> (-112.23, 5)
  line L178 (-112.23, 5) -> (-113.74, 5)
  line L179 (-113.74, 5) -> (-113.74, 0)
  line L180 (-41.885, 0) -> (-41.885, 5)
  line L181 (-41.885, 5) -> (-43.355, 5)
  line L182 (-43.355, 5) -> (-43.355, 12.5)
  line L183 (43.355, 12.5) -> (43.355, 5)
  line L184 (43.355, 5) -> (41.885, 5)
  line L185 (41.885, 5) -> (41.885, 0)
  line L186 (41.885, 0) -> (55.75, 0)
  line L187 (113.74, 0) -> (113.74, 5)
  line L188 (113.74, 5) -> (112.23, 5)
  line L189 (112.23, 5) -> (112.23, 12.5)
  line L190 (112.23, 12.5) -> (113.74, 12.5)
  line L191 (-113.74, 0) -> (-105.75, 0)
  dimension "d72" = 80
  dimension "d73" = 120
  dimension "d75" = 16.75
  dimension "d76" = 4
  dimension "d77" = 4
  dimension "d78" = 4
  dimension "d79" = 4
  dimension "d257" = 24.75
  measures "d73" distance of origin
  measures "d75" distance of origin L172
  measures "d76" diameter of A4
  measures "d77" diameter of A5
  measures "d78" diameter of A7
  measures "d79" diameter of A6
  measures "d257" distance of origin
extrude "Extrude5" cut sketch "Power holes" against normal through all contours A4 | A5 | A6 | A7
hole "Hole1" at (8, 117.5858, -119.1642) direction (-1, 0, 0) diameter 4 end up to surface (8 mm away)
hole "Hole2" at (8, 418.4142, -98.9142) direction (-1, 0, 0) diameter 4 end up to surface (8 mm away)
hole "Hole3" at (8, -1.4142, -107.1869) direction (-1, 0, 0) diameter 4 end up to surface (8 mm away)
hole "Hole4" at (8, 355.5858, 119.1642) direction (-1, 0, 0) diameter 4 end up to surface (8 mm away)
hole "Hole5" at (8, 236.5858, -119.1642) direction (-1, 0, 0) diameter 4 end up to surface (8 mm away)
hole "Hole6" at (8, 61.4142, 119.1642) direction (-1, 0, 0) diameter 4 end up to surface (8 mm away)
hole "Hole7" at (8, -1.4142, 107.1642) direction (-1, 0, 0) diameter 4 end up to surface (8 mm away)
hole "Hole8" at (8, 61.4142, -119.1642) direction (-1, 0, 0) diameter 4 end up to surface (8 mm away)
hole "Hole9" at (8, 355.5858, -119.1642) direction (-1, 0, 0) diameter 4 end up to surface (8 mm away)
hole "Hole10" at (8, 418.4142, 98.9142) direction (-1, 0, 0) diameter 4 end up to surface (8 mm away)
hole "Hole11" at (8, -1.4142, 54.3358) direction (-1, 0, 0) diameter 4 end up to surface (8 mm away)
hole "Hole12" at (8, 236.5858, 119.1642) direction (-1, 0, 0) diameter 4 end up to surface (8 mm away)
hole "Hole13" at (8, 299.4142, -119.1642) direction (-1, 0, 0) diameter 4 end up to surface (8 mm away)
hole "Hole14" at (8, 117.5858, 119.1642) direction (-1, 0, 0) diameter 4 end up to surface (8 mm away)
hole "Hole15" at (8, 180.4142, -119.1642) direction (-1, 0, 0) diameter 4 end up to surface (8 mm away)
hole "Hole16" at (8, -1.4142, -54.3358) direction (-1, 0, 0) diameter 4 end up to surface (8 mm away)
hole "Hole17" at (8, 180.4142, 119.1642) direction (-1, 0, 0) diameter 4 end up to surface (8 mm away)
hole "Hole18" at (8, 299.4142, 119.1642) direction (-1, 0, 0) diameter 4 end up to surface (8 mm away)
hole "Hole19" at (8, -1.4142, -26.4142) direction (-1, 0, 0) diameter 4 end up to surface (8 mm away)
hole "Hole20" at (8, -1.4142, 26.4142) direction (-1, 0, 0) diameter 4 end up to surface (8 mm away)
equation "pannel_thickness = 8 mm"
equation "d7 = pannel_thickness"
equation "d18 = Square_joint_thickness"
equation "d20 = pannel_thickness"
equation "d21 = pannel_thickness"
equation "d29 = pannel_thickness"
equation "d30 = pannel_thickness"
equation "d31 = tslo_diameter + 0.02 mm"
equation "d33 = ( ( 7 - 4 ) / 2 ) * 1 mm + 0.01 mm"
equation "d37 = tslo_diameter + 0.02 mm"
equation "d40 = ( ( 7 - 4 ) / 2 ) * 1 mm + 0.01 mm"
equation "d45 = ( ( 7 - 4 ) / 2 ) * 1 mm + 0.01 mm"
equation "d46 = tslo_diameter + 0.02 mm"
equation "d64 = ( 75 / 2 ) * 1 mm"
equation "d66 = tslo_diameter + 0.02 mm"
equation "d68 = ( ( 7 - 4 ) / 2 ) * 1 mm + 0.01 mm"
equation "d83 = pannel_thickness + 12 mm"
equation "d84 = pannel_thickness"
equation "d85 = pannel_thickness + 12 mm"
equation "tslo_diameter = 4 mm"
equation "Square_joint_thickness = 50 mm"
equation "dbToolDia = 4 mm"
equation "dbOffset = 0 mm" comment "Do NOT change formula"
equation "dbRadius = ( dbToolDia + dbOffset ) / 2" comment "Do NOT change formula"
equation "dbMinPercent = 10"
equation "dbHoleOffset = dbRadius / sqrt(2)" comment "Do NOT change formula"
equation "d264 = dbRadius * 2"
equation "d266 = dbHoleOffset"
equation "d267 = dbHoleOffset"
equation "d269 = dbRadius * 2"
equation "d271 = dbHoleOffset"
equation "d272 = dbHoleOffset"
equation "d274 = dbRadius * 2"
equation "d276 = dbHoleOffset"
equation "d277 = dbHoleOffset"
equation "d279 = dbRadius * 2"
equation "d281 = dbHoleOffset"
equation "d282 = dbHoleOffset"
equation "d284 = dbRadius * 2"
equation "d286 = dbHoleOffset"
equation "d287 = dbHoleOffset"
equation "d289 = dbRadius * 2"
equation "d291 = dbHoleOffset"
equation "d292 = dbHoleOffset"
equation "d294 = dbRadius * 2"
equation "d296 = dbHoleOffset"
equation "d297 = dbHoleOffset"
equation "d299 = dbRadius * 2"
equation "d301 = dbHoleOffset"
equation "d302 = dbHoleOffset"
equation "d304 = dbRadius * 2"
equation "d306 = dbHoleOffset"
equation "d307 = dbHoleOffset"
equation "d309 = dbRadius * 2"
equation "d311 = dbHoleOffset"
equation "d312 = dbHoleOffset"
equation "d314 = dbRadius * 2"
equation "d316 = dbHoleOffset"
equation "d317 = dbHoleOffset"
equation "d319 = dbRadius * 2"
equation "d321 = dbHoleOffset"
equation "d322 = dbHoleOffset"
equation "d324 = dbRadius * 2"
equation "d326 = dbHoleOffset"
equation "d327 = dbHoleOffset"
equation "d329 = dbRadius * 2"
equation "d331 = dbHoleOffset"
equation "d332 = dbHoleOffset"
equation "d334 = dbRadius * 2"
equation "d336 = dbHoleOffset"
equation "d337 = dbHoleOffset"
equation "d339 = dbRadius * 2"
equation "d341 = dbHoleOffset"
equation "d342 = dbHoleOffset"
equation "d344 = dbRadius * 2"
equation "d346 = dbHoleOffset"
equation "d347 = dbHoleOffset"
equation "d349 = dbRadius * 2"
equation "d351 = dbHoleOffset"
equation "d352 = dbHoleOffset"
equation "d354 = dbRadius * 2"
equation "d356 = dbHoleOffset"
equation "d357 = dbHoleOffset"
equation "d359 = dbRadius * 2"
equation "d361 = dbHoleOffset"
equation "d362 = dbHoleOffset"
